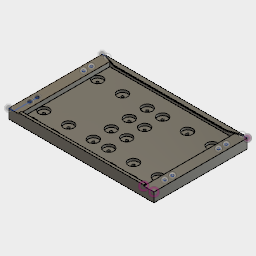
Tablet Mounts v6 (Autodesk Fusion 360 design; units mm, degrees)
Autodesk Fusion 360 part; units mm, degrees
sketch "Sketch1" plane through (0, 0, 0) normal (0, 1, 0) x (1, 0, 0)
  line L0 (-121.0529, -85.8521) -> (121.9471, -85.8521)
  line L1 (121.9471, -85.8521) -> (121.9471, 86.1479)
  line L2 (121.9471, 86.1479) -> (-121.0529, 86.1479)
  line L3 (-121.0529, 86.1479) -> (-121.0529, -85.8521)
  line L4 (-121.0529, -85.8521) -> (-121.0529, 86.1479)
  line L5 (121.9471, 86.1479) -> (-121.0529, 86.1479)
  line L6 (-121.0529, 86.1479) -> (-121.0529, 91.1479)
  line L7 (-121.0529, 91.1479) -> (121.9471, 91.1479)
  line L8 (121.9471, 91.1479) -> (121.9471, 86.1479)
  line L9 (-121.0529, -85.8521) -> (121.9471, -85.8521)
  line L10 (121.9471, -85.8521) -> (121.9471, -90.8521)
  line L11 (121.9471, -90.8521) -> (-121.0529, -90.8521)
  line L12 (-121.0529, -90.8521) -> (-121.0529, -85.8521)
  line L13 (121.9471, 86.1479) -> (136.9471, 86.1479)
  line L14 (136.9471, 86.1479) -> (136.9471, -85.8521)
  line L15 (136.9471, -85.8521) -> (121.9471, -85.8521)
  line L16 (121.9471, -85.8521) -> (121.9471, 86.1479)
  line L17 (-121.0529, 86.1479) -> (-136.0529, 86.1479)
  line L18 (-136.0529, 86.1479) -> (-136.0529, -85.8521)
  line L19 (-136.0529, -85.8521) -> (-121.0529, -85.8521)
  line L20 (-121.0529, -85.8521) -> (-121.0529, 86.1479)
  line L21 (-121.0529, 91.1479) -> (-136.0529, 91.1479)
  line L22 (-136.0529, 91.1479) -> (-136.0529, 86.1479)
  line L23 (-136.0529, 86.1479) -> (-121.0529, 86.1479)
  line L24 (-121.0529, 86.1479) -> (-121.0529, 91.1479)
  line L25 (-136.0529, -85.8521) -> (-121.0529, -85.8521)
  line L26 (-121.0529, -85.8521) -> (-121.0529, -90.8521)
  line L27 (-121.0529, -90.8521) -> (-136.0529, -90.8521)
  line L28 (-136.0529, -90.8521) -> (-136.0529, -85.8521)
  line L29 (136.9471, -85.8521) -> (121.9471, -85.8521)
  line L30 (121.9471, -85.8521) -> (121.9471, -90.8521)
  line L31 (121.9471, -90.8521) -> (136.9471, -90.8521)
  line L32 (136.9471, -90.8521) -> (136.9471, -85.8521)
  line L33 (121.9471, 91.1479) -> (136.9471, 91.1479)
  line L34 (136.9471, 91.1479) -> (136.9471, 86.1479)
  line L35 (136.9471, 86.1479) -> (121.9471, 86.1479)
  line L36 (121.9471, 86.1479) -> (121.9471, 91.1479)
extrude "Extrude1" add sketch "Sketch1" along normal blind 8 contours L0 L1 L2 L3 L4 L5 L9 L16 L20 makes body 1
extrude "Extrude2" add sketch "Sketch1" along normal blind 16.6 separate body contours L3 L4 L17 L18 L19 L20 L23 L25 | L0 L9 L10 L11 L12 L26 L30 | L12 L19 L25 L26 L27 L28 | L10 L15 L29 L30 L31 L32 | L1 L13 L14 L15 L16 L29 L35 | L2 L5 L6 L7 L8 L24 L36 | L6 L17 L21 L22 L23 L24 | L8 L13 L33 L34 L35 L36 makes body 2
sketch "Top Lid" plane through (0, 16.6, 0) normal (0, 1, 0) x (-1, 0, 0)
  line L0 (-121.9471, -86.1479) -> (-121.9471, 85.8521)
  line L1 (-121.9471, 85.8521) -> (121.0529, 85.8521)
  line L2 (121.0529, 85.8521) -> (121.0529, -86.1479)
  line L3 (121.0529, -86.1479) -> (-121.9471, -86.1479)
  line L4 (-136.9471, -91.1479) -> (136.0529, -91.1479)
  line L5 (136.0529, -91.1479) -> (136.0529, 90.8521)
  line L6 (136.0529, 90.8521) -> (-136.9471, 90.8521)
  line L7 (-136.9471, 90.8521) -> (-136.9471, -91.1479)
  line L8 (-136.9471, -91.1479) -> (-121.9471, -86.1479)
  line L9 (-121.9471, -86.1479) -> (-109.9471, -82.1479)
  line L10 (136.0529, -91.1479) -> (121.0529, -86.1479)
  line L11 (121.0529, -86.1479) -> (109.0529, -82.1479)
  line L12 (109.0529, -82.1479) -> (-109.9471, -82.1479)
  line L13 (136.0529, -91.1479) -> (-136.9471, -91.1479)
extrude "Extrude3" add sketch "Top Lid" along normal blind 2 separate body contours L3 L9 L11 L12 | L3 L4 L8 L10 L13 makes body 3
sketch "Sketch3" plane through (0, 16.6, 0) normal (0, 1, 0) x (-1, 0, 0)
  line L0 (-121.9471, -86.1479) -> (-121.9471, 85.8521)
  line L1 (-121.9471, 85.8521) -> (121.0529, 85.8521)
  line L2 (121.0529, 85.8521) -> (121.0529, -86.1479)
  line L3 (121.0529, -86.1479) -> (-121.9471, -86.1479)
  line L4 (-136.9471, -91.1479) -> (136.0529, -91.1479)
  line L5 (136.0529, -91.1479) -> (136.0529, 90.8521)
  line L6 (136.0529, 90.8521) -> (-136.9471, 90.8521)
  line L7 (-136.9471, 90.8521) -> (-136.9471, -91.1479)
  line L8 (121.0529, 85.8521) -> (-122.0581, 85.8521)
  line L9 (-122.0581, 85.8521) -> (-122.0581, 90.8521)
  line L10 (-122.0581, 90.8521) -> (121.0529, 90.8521)
  line L11 (121.0529, 90.8521) -> (121.0529, 85.8521)
extrude "Extrude4" add sketch "Sketch3" along normal blind 2 contours L1 L6 L8 L9 L10 L11 bodies 2
sketch "Tab Wall" plane through (0, 0, 85.8521) normal (0, 0, -1) x (-1, 0, 0)
  line L0 (-121.9471, 0) -> (121.0529, 0)
  line L1 (121.0529, 0) -> (121.0529, 16.6)
  line L2 (121.0529, 16.6) -> (121.0529, 18.6)
  line L3 (121.0529, 18.6) -> (-122.0581, 18.6)
  line L4 (-122.0581, 18.6) -> (-122.0581, 16.6)
  line L5 (-122.0581, 16.6) -> (-121.9471, 16.6)
  line L6 (-121.9471, 16.6) -> (-121.9471, 0)
  line L7 (-122.0581, 18.6) -> (121.0529, 18.6)
  line L8 (121.0529, 18.6) -> (121.0529, 16.6)
  line L9 (121.0529, 16.6) -> (-122.0581, 16.6)
  line L10 (-122.0581, 16.6) -> (-122.0581, 18.6)
  line L11 (-122.0581, 18.6) -> (-102.0581, 18.6)
  line L12 (-102.0581, 18.6) -> (-92.0581, 18.6)
  line L13 (-92.0581, 18.6) -> (-92.0581, 16.6)
  line L14 (-92.0581, 16.6) -> (-102.0581, 16.6)
  line L15 (-102.0581, 16.6) -> (-102.0581, 18.6)
  line L16 (121.0529, 18.6) -> (101.0529, 18.6)
  line L17 (101.0529, 18.6) -> (91.0529, 18.6)
  line L18 (91.0529, 18.6) -> (91.0529, 16.6)
  line L19 (91.0529, 16.6) -> (101.0529, 16.6)
  line L20 (101.0529, 16.6) -> (101.0529, 18.6)
  line L21 (-92.0581, 18.6) -> (-62.0581, 18.6)
  line L22 (-62.0581, 18.6) -> (-52.0581, 18.6)
  line L23 (-52.0581, 18.6) -> (-52.0581, 16.6)
  line L24 (-52.0581, 16.6) -> (-62.0581, 16.6)
  line L25 (-62.0581, 16.6) -> (-62.0581, 18.6)
  line L26 (91.0529, 18.6) -> (61.0529, 18.6)
  line L27 (61.0529, 18.6) -> (51.0529, 18.6)
  line L28 (51.0529, 18.6) -> (51.0529, 16.6)
  line L29 (51.0529, 16.6) -> (61.0529, 16.6)
  line L30 (61.0529, 16.6) -> (61.0529, 18.6)
  dimension "d22" = 20
  dimension "d23" = 10
  dimension "d24" = 20
  dimension "d25" = 10
  dimension "d26" = 30
  dimension "d27" = 10
  dimension "d28" = 30
  dimension "d29" = 10
  measures "d22" distance of L3.end L11.end
  measures "d23" distance of L11.end L12.end
  measures "d24" distance of L2.end L16.end
  measures "d25" distance of L16.end L17.end
  measures "d26" distance of L12.end L21.end
  measures "d27" distance of L21.end L22.end
  measures "d28" distance of L17.end L26.end
  measures "d29" distance of L26.end L27.end
extrude "Extrude5" add sketch "Tab Wall" along normal blind 2 separate body contours L3 L7 L9 L12 L13 L14 L15 | L3 L7 L9 L17 L18 L19 L20 | L3 L7 L9 L22 L23 L24 L25 | L3 L7 L9 L27 L28 L29 L30 makes body 4 at (55.3914, 18.6, 84.5188) makes body 5 at (-57.7196, 16.6, 84.5188) makes body 6 at (95.3914, 18.6, 84.5188) makes body 7 at (-97.7196, 16.6, 84.5188)
chamfer "Chamfer1" distance 1 angle 45 1 edges at (97.0581, 18.6, 83.8521) on bodies 6
chamfer "Chamfer2" distance 1 angle 45 7 edges at (-56.0529, 18.6, 83.8521) (-56.0529, 16.6, 83.8521) (97.0581, 16.6, 83.8521) (-96.0529, 18.6, 83.8521) (-96.0529, 16.6, 83.8521) (57.0581, 18.6, 83.8521) (57.0581, 16.6, 83.8521) on bodies 4 5 6 7
extrude "Extrude6" add 1 faces at (131.9471, 0, -28.8145) along direction (0, -1, 0) blind 2 on bodies 2 bodies 2 1
extrude "Extrude7" add 1 faces at (-40.0529, 0, -28.8145) along direction (0, -1, 0) blind 2 on bodies 2 bodies 2
sketch "Bottom Inner" plane through (0, 8, 0) normal (0, 1, 0) x (-1, 0, 0)
  line L0 (-121.9471, 85.8521) -> (-121.9471, -86.1479)
  line L1 (-121.9471, -86.1479) -> (121.0529, -86.1479)
  line L2 (121.0529, -86.1479) -> (121.0529, 85.8521)
  line L3 (121.0529, 85.8521) -> (-121.9471, 85.8521)
  line L4 (121.0529, -86.1479) -> (121.0529, -52.6479)
  line L5 (121.0529, -52.6479) -> (121.0529, -17.6479)
  line L6 (121.0529, -17.6479) -> (121.0529, 17.3521)
  line L7 (121.0529, 17.3521) -> (121.0529, 52.3521)
  line L8 (121.0529, 52.3521) -> (121.0529, 85.8521)
  line L9 (121.0529, -86.1479) -> (111.0529, -86.1479)
  line L10 (111.0529, -86.1479) -> (62.8029, -86.1479)
  line L11 (62.8029, -86.1479) -> (14.5529, -86.1479)
  line L12 (14.5529, -86.1479) -> (-15.4471, -86.1479)
  line L13 (-15.4471, -86.1479) -> (-63.6971, -86.1479)
  line L14 (-63.6971, -86.1479) -> (-111.9471, -86.1479)
  line L15 (-111.9471, -86.1479) -> (-121.9471, -86.1479)
  circle A0 centre (111.0529, -52.6479) radius 10
  circle A1 centre (62.8029, -52.6479) radius 10
  circle A2 centre (14.5529, -52.6479) radius 10
  circle A3 centre (-15.4471, -52.6479) radius 10
  circle A4 centre (-63.6971, -52.6479) radius 10
  circle A5 centre (-111.9471, -52.6479) radius 10
  circle A6 centre (14.5529, -17.6479) radius 10
  circle A7 centre (14.5529, 17.3521) radius 10
  circle A8 centre (14.5529, 52.3521) radius 10
  circle A9 centre (62.8029, 52.3521) radius 10
  circle A10 centre (111.0529, 52.3521) radius 10
  circle A11 centre (-15.4471, 52.3521) radius 10
  circle A12 centre (-63.6971, 52.3521) radius 10
  circle A13 centre (-111.9471, 52.3521) radius 10
  circle A14 centre (-15.4471, -17.6479) radius 10
  circle A15 centre (-15.4471, 17.3521) radius 10
  dimension "d43" = 10
  dimension "d44" = 48.25
  dimension "d45" = 48.25
  dimension "d46" = 30
  dimension "d47" = 48.25
  dimension "d48" = 48.25
  dimension "d49" = 20
  dimension "d50" = 20
  dimension "d51" = 20
  dimension "d52" = 20
  dimension "d53" = 20
  dimension "d54" = 20
  dimension "d55" = 20
  dimension "d56" = 20
  dimension "d57" = 20
  dimension "d58" = 20
  dimension "d59" = 20
  dimension "d60" = 20
  dimension "d61" = 20
  dimension "d62" = 20
  dimension "d63" = 20
  dimension "d64" = 20
  measures "d43" distance of L1.end L9.end
  measures "d44" distance of L9.end L10.end
  measures "d45" distance of L10.end L11.end
  measures "d46" distance of L11.end L12.end
  measures "d47" distance of L12.end L13.end
  measures "d48" distance of L13.end L14.end
  measures "d49" diameter of A0
  measures "d50" diameter of A1
  measures "d51" diameter of A2
  measures "d52" diameter of A3
  measures "d53" diameter of A4
  measures "d54" diameter of A5
  measures "d55" diameter of A6
  measures "d56" diameter of A7
  measures "d57" diameter of A8
  measures "d58" diameter of A9
  measures "d59" diameter of A10
  measures "d60" diameter of A11
  measures "d61" diameter of A12
  measures "d62" diameter of A13
  measures "d63" diameter of A14
  measures "d64" diameter of A15
extrude "Extrude8" cut sketch "Bottom Inner" against normal blind 4.5 contours A13 | A5 | A0 | A10 | A1 | A2 | A3 | A4 | A6 | A7 | A8 | A9 | A11 | A12 | A14 | A15 bodies 2
sketch "Sketch6" plane through (0, 3.5, 0) normal (0, 1, 0) x (-1, 0, 0)
  circle A0 centre (111.0529, -52.6479) radius 10
  circle A1 centre (111.0529, -52.6479) radius 2.385
  dimension "d67" = 4.77
  measures "d67" diameter of A1
extrude "Extrude9" cut sketch "Sketch6" against normal blind 20 contours A1 bodies 2
sketch "Sketch7" plane through (0, 3.5, 0) normal (0, 1, 0) x (-1, 0, 0)
  circle A0 centre (62.8029, -52.6479) radius 10
  circle A1 centre (62.8029, -52.6479) radius 2.385
  dimension "d70" = 4.77
  measures "d70" diameter of A1
extrude "Extrude10" cut sketch "Sketch7" against normal blind 20 contours A1 bodies 2
sketch "Sketch8" plane through (0, 3.5, 0) normal (0, 1, 0) x (-1, 0, 0)
  circle A0 centre (14.5529, -52.6479) radius 10
  circle A1 centre (14.5529, -52.6479) radius 2.385
  dimension "d73" = 4.77
  measures "d73" diameter of A1
extrude "Extrude11" cut sketch "Sketch8" against normal blind 22 contours A1 bodies 2
sketch "Sketch9" plane through (0, 3.5, 0) normal (0, 1, 0) x (-1, 0, 0)
  circle A0 centre (-15.4471, -52.6479) radius 10
  circle A1 centre (-15.4471, -52.6479) radius 2.385
  dimension "d76" = 4.77
  measures "d76" diameter of A1
extrude "Extrude12" cut sketch "Sketch9" against normal blind 20 contours A1 bodies 2
sketch "Sketch10" plane through (0, 3.5, 0) normal (0, 1, 0) x (-1, 0, 0)
  circle A0 centre (-63.6971, -52.6479) radius 10
  circle A1 centre (-63.6971, -52.6479) radius 2.385
  dimension "d79" = 4.77
  measures "d79" diameter of A1
extrude "Extrude13" cut sketch "Sketch10" against normal blind 20 contours A1 bodies 2
sketch "Sketch11" plane through (0, 3.5, 0) normal (0, 1, 0) x (-1, 0, 0)
  circle A0 centre (-111.9471, -52.6479) radius 10
  circle A1 centre (-111.9471, -52.6479) radius 2.385
  dimension "d82" = 4.77
  measures "d82" diameter of A1
extrude "Extrude14" cut sketch "Sketch11" against normal blind 20 contours A1 bodies 2
sketch "Sketch12" plane through (0, 3.5, 0) normal (0, 1, 0) x (-1, 0, 0)
  circle A0 centre (14.5529, -17.6479) radius 10
  circle A1 centre (14.5529, -17.6479) radius 2.385
  dimension "d85" = 4.77
  measures "d85" diameter of A1
extrude "Extrude15" cut sketch "Sketch12" against normal blind 20 contours A1 bodies 2
sketch "Sketch13" plane through (0, 0, 0) normal (0, 1, 0) x (1, 0, 0)
sketch "Sketch14" plane through (0, 3.5, 0) normal (0, 1, 0) x (-1, 0, 0)
  circle A0 centre (-15.4471, -17.6479) radius 10
  circle A1 centre (-15.4471, -17.6479) radius 2.385
  dimension "d88" = 4.77
  measures "d88" diameter of A1
extrude "Extrude16" cut sketch "Sketch14" against normal blind 20 contours A1 bodies 2
sketch "Sketch15" plane through (0, 3.5, 0) normal (0, 1, 0) x (-1, 0, 0)
  circle A0 centre (14.5529, 17.3521) radius 10
  circle A1 centre (14.5529, 17.3521) radius 2.385
  dimension "d91" = 4.77
  measures "d91" diameter of A1
extrude "Extrude17" cut sketch "Sketch15" against normal blind 20 contours A1 bodies 2
sketch "Sketch16" plane through (0, 3.5, 0) normal (0, 1, 0) x (-1, 0, 0)
  circle A0 centre (-15.4471, 17.3521) radius 10
  circle A1 centre (-15.4471, 17.3521) radius 2.385
  dimension "d94" = 4.77
  measures "d94" diameter of A1
extrude "Extrude18" cut sketch "Sketch16" against normal blind 20 contours A1 bodies 2
sketch "Sketch17" plane through (0, 3.5, 0) normal (0, 1, 0) x (-1, 0, 0)
  circle A0 centre (-15.4471, 52.3521) radius 10
  circle A1 centre (-15.4471, 52.3521) radius 2.385
  dimension "d97" = 4.77
  measures "d97" diameter of A1
extrude "Extrude19" cut sketch "Sketch17" against normal blind 20 contours A1 bodies 2
sketch "Sketch18" plane through (0, 3.5, 0) normal (0, 1, 0) x (-1, 0, 0)
  circle A0 centre (14.5529, 52.3521) radius 10
  circle A1 centre (14.5529, 52.3521) radius 2.385
  dimension "d100" = 4.77
  measures "d100" diameter of A1
extrude "Extrude20" cut sketch "Sketch18" against normal blind 20 contours A1 bodies 2
sketch "Sketch19" plane through (0, 3.5, 0) normal (0, 1, 0) x (-1, 0, 0)
  circle A0 centre (62.8029, 52.3521) radius 10
  circle A1 centre (62.8029, 52.3521) radius 2.385
  dimension "d103" = 4.77
  measures "d103" diameter of A1
extrude "Extrude21" cut sketch "Sketch19" against normal blind 20 contours A1 bodies 2
sketch "Sketch20" plane through (0, 3.5, 0) normal (0, 1, 0) x (-1, 0, 0)
  circle A0 centre (111.0529, 52.3521) radius 10
  circle A1 centre (111.0529, 52.3521) radius 2.385
  dimension "d106" = 4.77
  measures "d106" diameter of A1
extrude "Extrude22" cut sketch "Sketch20" against normal blind 20 contours A1 bodies 2
sketch "Sketch21" plane through (0, 3.5, 0) normal (0, 1, 0) x (-1, 0, 0)
  circle A0 centre (-63.6971, 52.3521) radius 10
  circle A1 centre (-63.6971, 52.3521) radius 2.385
  dimension "d109" = 4.77
  measures "d109" diameter of A1
extrude "Extrude23" cut sketch "Sketch21" against normal blind 20 contours A1 bodies 2
sketch "Sketch22" plane through (0, 3.5, 0) normal (0, 1, 0) x (-1, 0, 0)
  circle A0 centre (-111.9471, 52.3521) radius 10
  circle A1 centre (-111.9471, 52.3521) radius 2.385
  dimension "d112" = 4.77
  measures "d112" diameter of A1
extrude "Extrude24" cut sketch "Sketch22" against normal blind 20 contours A1 bodies 2
extrude "Extrude25" add 1 faces at (-136.0529, 10.4, -30.4812) along direction (-1, 0, 0) blind 5 on bodies 2 bodies 2 3
extrude "Extrude26" add 1 faces at (136.9471, 10.4, -30.4812) along direction (1, 0, 0) blind 5 on bodies 2 bodies 2
sketch "Sketch23" plane through (0, 16.6, 0) normal (0, 1, 0) x (-1, 0, 0)
  line L0 (121.0529, -86.1479) -> (136.0529, -91.1479)
  line L1 (136.0529, -91.1479) -> (141.0529, -91.1479)
  line L2 (141.0529, -91.1479) -> (141.0529, 90.8521)
  line L3 (141.0529, 90.8521) -> (121.0529, 90.8521)
  line L4 (121.0529, 90.8521) -> (121.0529, 85.8521)
  line L5 (121.0529, 85.8521) -> (121.0529, -86.1479)
  line L6 (141.0529, -91.1479) -> (131.0529, -91.1479)
  circle A0 centre (131.0529, -60.1479) radius 2.385
  circle A1 centre (131.0529, -45.1479) radius 2.385
  line L7 (141.0529, 90.8521) -> (131.0529, 90.8521)
  line L8 (131.0529, 90.8521) -> (131.0529, 59.8521)
  line L9 (131.0529, 59.8521) -> (131.0529, 44.8521)
  circle A2 centre (131.0529, 59.8521) radius 2.385
  circle A3 centre (131.0529, 44.8521) radius 2.385
  line L10 (-122.0581, 90.8521) -> (-141.9471, 90.8521)
  circle A4 centre (-132.0026, 59.8521) radius 2.385
  circle A5 centre (-132.0026, 44.8521) radius 2.385
  line L11 (-141.9471, -91.1479) -> (-131.9471, -91.1479)
  circle A6 centre (-131.9471, -45.1479) radius 2.385
  circle A7 centre (-131.9471, -60.1479) radius 2.385
  point P0 (-141.9471, -91.1479)
  dimension "d119" = 10
  dimension "d126" = 4.77
  dimension "d127" = 4.77
  dimension "d128" = 10
  dimension "d129" = 31
  dimension "d130" = 15
  dimension "d131" = 4.77
  dimension "d132" = 4.77
  dimension "d135" = 4.77
  dimension "d136" = 4.77
  dimension "d140" = 4.77
  dimension "d141" = 4.77
  measures "d119" distance of L1.end L6.end
  measures "d126" diameter of A0
  measures "d127" diameter of A1
  measures "d128" distance of L2.end L7.end
  measures "d129" distance of L7.end L8.end
  measures "d130" distance of L8.end L9.end
  measures "d131" diameter of A2
  measures "d132" diameter of A3
  measures "d135" diameter of A4
  measures "d136" diameter of A5
  measures "d140" diameter of A6
  measures "d141" diameter of A7
extrude "Extrude27" cut sketch "Sketch23" against normal blind 20 contours A0 | A1 | L8 L9 A2 | L8 L9 A2 | A3 bodies 2
extrude "Extrude28" cut sketch "Sketch23" against normal blind 20 contours A4 | A5 | A6 | A7 bodies 2
equation "d14 = 8 mm + 8.6 mm"
